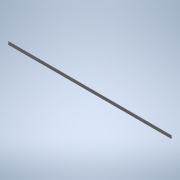
# Autodesk Inventor part: SP55V1 Chapa Guia
Saved by Autodesk Inventor 2021.2 (Build 252289000, 289)
## iProperties
Created: 2026-10-05
Part Number: SP55V1 Chapa Guia
Material: Generic
Document SubType Name: Sheet Metal
Designer: nelso
Density: 1 g/cm^3
Sheet Metal Rule: Default_mm
Appearance: Default
Author: nelso
Autodesk Inventor part; units mm, degrees
ref_plane "YZ Plane" through (0, 0, 0) normal (1, 0, 0) x (0, 1, 0)
ref_plane "XZ Plane" through (0, 0, 0) normal (0, 1, 0) x (-1, 0, 0)
ref_plane "XY Plane" through (0, 0, 0) normal (0, 0, 1) x (1, 0, 0)
sketch "Sketch1" plane through (0, 0, 0) normal (0, 1, 0) x (-1, 0, 0)
  line L0 (870, 16) -> (-870, 16)
  line L1 (-870, 16) -> (-870, -16)
  line L2 (-870, -16) -> (870, -16)
  line L3 (870, -16) -> (870, 16)
  line L4 (870, 16) -> (-870, -16) construction
  line L5 (-870, 16) -> (870, -16) construction
  point P0 (0, 0)
  dimension "d0" = 1740
  dimension "d1" = 32
  measures "d0" distance of L2.end L1.end
  measures "d1" distance of L1.end L0.end
extrude "Plate1" add sketch "Sketch1" along normal blind 3.2
sketch "Sketch3" plane through (0, 3.2, 0) normal (0, 1, 0) x (1, 0, 0)
  line L0 (0, 0) -> (-700, 0)
  line L1 (0, 0) -> (0, 5)
  point P0 (700, 0)
  dimension "d13" = 700
  dimension "d14" = 5
  constraints: 4 end point, 2 coincident, 1 horizontal, 1 symmetric about line, 1 vertical
  measures "d13" distance of L0.start L0.end
  measures "d14" distance of L0.start L1.end
hole "Hole1" at (0, 3.2, 0) at (-700, 3.2, 0) at (700, 3.2, 0) direction (0, -1, 0) diameter 4.5 depth 3.2 clearance for "Countersunk Flat Head Screw ISO 2009/7046" size "M4" standard "ISO"
fillet "Corner Round1" radius 3 4 edges at (870, 1.6, 16) (-870, 1.6, 16) (870, 1.6, -16) (-870, 1.6, -16)
equation "\"d20\" = Thickness"
equation "\"d2\" = Thickness"
equation "\"BendReliefWidth\" = Thickness"
equation "\"BendReliefDepth\" = 0.5 * Thickness"
equation "\"CornerReliefSize\" = 4 * Thickness"
equation "\"MinimumRemnant\" = 2 * Thickness"
equation "\"TransitionRadius\" = BendRadius"
equation "\"JacobiRadiusSize\" = BendRadius"
equation "\"GapSize\" = Thickness"
equation "\"Thickness\" = 3.2"
equation "\"BendRadius\" = 1.516"
body "Solid1"
